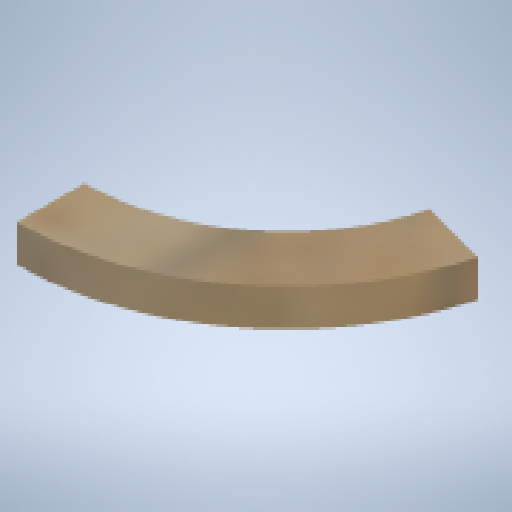
# Autodesk Inventor part: gear_plate_cover_3
Saved by Autodesk Inventor 2026.1 (Build 301233020, 233B)
## iProperties
Created: 2025-11-01
Part Number: gear_plate_cover_3
Material: 木材 (カエデ材)
Document SubType Name: Modeling
Designer: hibik
Density: 0.67 g/cm^3
Appearance: ナチュラル カエデ材 - 光沢 濃い着色
Author: hibik
Autodesk Inventor part; units mm, degrees
ref_plane "YZ Plane" through (0, 0, 0) normal (1, 0, 0) x (0, 1, 0)
ref_plane "XZ Plane" through (0, 0, 0) normal (0, 1, 0) x (-1, 0, 0)
ref_plane "XY Plane" through (0, 0, 0) normal (0, 0, 1) x (1, 0, 0)
sketch "スケッチ1" plane through (0, 0, 0) normal (0, 1, 0) x (-1, 0, 0)
  circle A0 centre (0, 0) radius 40
  circle A1 centre (0, 0) radius 30
  line L0 (0, 0) -> (0, 40)
  line L1 (0, 0) -> (-38.637, 10.3528)
  point P0 (-28.9778, 7.7646)
  point P1 (0, 30)
  dimension "d0" = 60
  dimension "d1" = 10
  dimension "d2" = 75
  constraints: 4 end point, 2 centre point, 2 coincident, 2 point on circle, 1 vertical
  measures "d0" diameter of A1
  measures "d1" radial gap between concentric circles of A0 A1
  measures "d2" angle of L0 L1
extrude "押し出し1" add sketch "スケッチ1" along normal blind 5.5 contours L0 A1 L1 A0 picked at (-10.6852, 34.8643)
